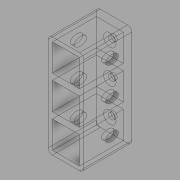
# Autodesk Inventor part: AK-C-C39-Holder
Saved by Autodesk Inventor 2016 (Build 200138000, 138)
## iProperties
Created: 2016-04-02
Part Number: AK-C-C39-Holder
Material: ABS Plastic
Document SubType Name: Modeling
Designer: admin
Density: 1.06 g/cm^3
Appearance: Smooth - White
Author: admin
Autodesk Inventor part; units mm, degrees
ref_plane "YZ Plane" through (0, 0, 0) normal (1, 0, 0) x (0, 1, 0)
ref_plane "XZ Plane" through (0, 0, 0) normal (0, 1, 0) x (-1, 0, 0)
ref_plane "XY Plane" through (0, 0, 0) normal (0, 0, 1) x (1, 0, 0)
derived "AK-C-C39-Main-Board.ipt"
sketch "Sketch2" plane through (0, 0, 0) normal (0, 1, 0) x (-1, 0, 0)
  line L0 (51.25, -29) -> (44, -29)
  line L1 (43.25, -29.75) -> (43.25, -31)
  line L2 (43.25, -31) -> (6.5, -31)
  line L3 (6.5, -31) -> (6.5, -29.75)
  line L4 (5.75, -29) -> (-5.75, -29)
  line L5 (-6.5, -29.75) -> (-6.5, -31)
  line L6 (-6.5, -31) -> (-43.25, -31)
  line L7 (-43.25, -31) -> (-43.25, -29.75)
  line L8 (-44, -29) -> (-51.25, -29)
  line L9 (-51.25, -29) -> (-53.75, -26.5)
  line L10 (-53.75, -26.5) -> (-53.75, -5.5)
  line L11 (-53.75, -5.5) -> (-56.25, -3)
  line L12 (-56.25, -3) -> (-56.25, 18)
  line L13 (-56.25, 18) -> (-54.5, 18)
  line L14 (-53.75, 18.75) -> (-53.75, 26.5)
  line L15 (-53.75, 26.5) -> (-51.25, 29)
  line L16 (-51.25, 29) -> (-44, 29)
  line L17 (-43.25, 29.75) -> (-43.25, 31)
  line L18 (-43.25, 31) -> (-6.5, 31)
  line L19 (-6.5, 31) -> (-6.5, 29.75)
  line L20 (-5.75, 29) -> (5.75, 29)
  line L21 (6.5, 29.75) -> (6.5, 31)
  line L22 (43.25, 31) -> (43.25, 29.75)
  line L23 (43.25, 31) -> (6.5, 31)
  line L24 (44, 29) -> (51.25, 29)
  line L25 (51.25, 29) -> (53.75, 26.5)
  line L26 (53.75, 26.5) -> (53.75, 18.75)
  line L27 (54.5, 18) -> (56.25, 18)
  line L28 (56.25, 18) -> (56.25, -3)
  line L29 (56.25, -3) -> (53.75, -5.5)
  line L30 (53.75, -5.5) -> (53.75, -26.5)
  line L31 (53.75, -26.5) -> (51.25, -29)
  line L32 (44.7, -32.225) -> (5, -32.225)
  line L33 (5, -32.225) -> (5, -29.925)
  line L34 (5, -29.925) -> (3, -29.925)
  line L35 (44.7, -29.925) -> (44.7, -32.225)
  line L36 (46.7, -29.925) -> (44.7, -29.925)
  line L37 (52.7, -29.3928) -> (52.7, -31.925)
  arc A0 (53.5536, -29.0392) -> (52.7, -29.3928) centre (53.2, -29.3928) ccw
  arc A1 (54.9678, -27.125) -> (54.6142, -27.9786) centre (54.9678, -27.625) ccw
  line L38 (55, -17.425) -> (55, -25.125)
  line L39 (0, -20.0068) -> (0, 12.0803) construction
  line L40 (33.1179, 0) -> (-42.957, 0) construction
  line L41 (57.8, 19.125) -> (57.8, -3.3607)
  line L42 (57.8, -3.3607) -> (55, -7.6074)
  line L43 (55.5, 19.125) -> (57.8, 19.125)
  line L44 (55.5, 29.925) -> (49.0175, 23.4425) construction
  line L45 (25.75, -24.5) -> (12.75, -24.5)
  line L46 (12.75, 24.5) -> (25.75, 24.5)
  line L47 (3.3524, -20) -> (-16.6476, -20)
  line L48 (-16.6476, -20) -> (-16.6476, 20)
  line L49 (-16.6476, 20) -> (3.3524, 20)
  line L50 (3.3524, 20) -> (3.3524, -20)
  line L51 (-23.9878, -15) -> (-31.9878, -15) construction
  line L52 (-31.9878, -15) -> (-31.9878, -7) construction
  line L53 (-31.9878, -7) -> (-23.9878, -7) construction
  line L54 (-23.9878, -7) -> (-23.9878, -15) construction
  line L55 (-34.9878, -15) -> (-42.9878, -15) construction
  line L56 (-42.9878, -15) -> (-42.9878, -7) construction
  line L57 (-42.9878, -7) -> (-34.9878, -7) construction
  line L58 (-34.9878, -7) -> (-34.9878, -15) construction
  line L59 (-23.9878, -4) -> (-31.9878, -4) construction
  line L60 (-31.9878, -4) -> (-31.9878, 4) construction
  line L61 (-31.9878, 4) -> (-23.9878, 4) construction
  line L62 (-23.9878, 4) -> (-23.9878, -4) construction
  line L63 (-34.9878, -4) -> (-42.9878, -4) construction
  line L64 (-42.9878, -4) -> (-42.9878, 4) construction
  line L65 (-42.9878, 4) -> (-34.9878, 4) construction
  line L66 (-34.9878, 4) -> (-34.9878, -4) construction
  line L67 (-23.9878, 7) -> (-31.9878, 7) construction
  line L68 (-31.9878, 7) -> (-31.9878, 15) construction
  line L69 (-31.9878, 15) -> (-23.9878, 15) construction
  line L70 (-23.9878, 15) -> (-23.9878, 7) construction
  line L71 (-34.9878, 7) -> (-42.9878, 7) construction
  line L72 (-42.9878, 7) -> (-42.9878, 15) construction
  line L73 (-42.9878, 15) -> (-34.9878, 15) construction
  line L74 (-34.9878, 15) -> (-34.9878, 7) construction
  line L75 (25.75, -22.5) -> (12.75, -22.5) construction
  line L76 (12.75, -22.5) -> (12.75, -9.5) construction
  line L77 (12.75, -9.5) -> (25.75, -9.5) construction
  line L78 (25.75, -9.5) -> (25.75, -22.5) construction
  line L79 (25.75, -6.5) -> (12.75, -6.5) construction
  line L80 (12.75, -6.5) -> (12.75, 6.5) construction
  line L81 (12.75, 6.5) -> (25.75, 6.5) construction
  line L82 (25.75, 6.5) -> (25.75, -6.5) construction
  line L83 (25.75, 9.5) -> (12.75, 9.5) construction
  line L84 (12.75, 9.5) -> (12.75, 22.5) construction
  line L85 (12.75, 22.5) -> (25.75, 22.5) construction
  line L86 (25.75, 22.5) -> (25.75, 9.5) construction
  line L87 (31.9633, -16) -> (17.7262, -16) construction
  line L88 (31.9633, 16) -> (18.8213, 16) construction
  line L89 (19.25, -23.7063) -> (19.25, 24.6931) construction
  arc A2 (10.75, -22.5) -> (12.75, -24.5) centre (12.75, -22.5) ccw
  arc A3 (25.75, -24.5) -> (27.75, -22.5) centre (25.75, -22.5) ccw
  arc A4 (12.75, 24.5) -> (10.75, 22.5) centre (12.75, 22.5) ccw
  arc A5 (27.75, 22.5) -> (25.75, 24.5) centre (25.75, 22.5) ccw
  line L90 (55, -25.125) -> (-54.9956, -25.125) construction
  line L91 (55.5, 25.125) -> (55.5, 23.125)
  line L92 (57.5, 25.125) -> (55.5, 25.125)
  line L93 (-57.5, 25.125) -> (-55.5, 25.125)
  line L94 (-55.5, 25.125) -> (-55.5, 23.125)
  line L95 (-57.5, -25.125) -> (-55, -25.125)
  line L96 (-55, -25.125) -> (-55, -17.425)
  line L97 (55, -25.125) -> (57.5, -25.125)
  line L98 (55.5, 25.125) -> (-55.5, 25.125) construction
  line L99 (48.25, -6.5) -> (48.25, 6.5)
  line L100 (50, -6.5) -> (50, 6.5)
  line L101 (50, -8) -> (48.25, -8)
  line L102 (50, 8) -> (48.25, 8)
  arc A6 (50, -8) -> (50, -6.5) centre (50, -7.25) ccw
  arc A7 (48.25, -6.5) -> (48.25, -8) centre (48.25, -7.25) ccw
  arc A8 (50, 6.5) -> (50, 8) centre (50, 7.25) ccw
  arc A9 (48.25, 8) -> (48.25, 6.5) centre (48.25, 7.25) ccw
  line L103 (-47.75, -6.5) -> (-47.75, 6.5)
  line L104 (-49.5, 8) -> (-47.75, 8)
  line L105 (-49.5, 6.5) -> (-49.5, -6.5)
  line L106 (-49.5, -8) -> (-47.75, -8)
  arc A10 (-47.75, -8) -> (-47.75, -6.5) centre (-47.75, -7.25) ccw
  arc A11 (-49.5, -6.5) -> (-49.5, -8) centre (-49.5, -7.25) ccw
  arc A12 (-47.75, 6.5) -> (-47.75, 8) centre (-47.75, 7.25) ccw
  arc A13 (-49.5, 8) -> (-49.5, 6.5) centre (-49.5, 7.25) ccw
  line L107 (43.75, -27) -> (35.5, -27)
  line L108 (33.75, -27) -> (33.75, -25.25)
  line L109 (35.5, -25.25) -> (43.75, -25.25)
  line L110 (-11, -27) -> (-19.25, -27)
  line L111 (-19.25, -25.25) -> (-11, -25.25)
  line L112 (-9.25, -25.25) -> (-9.25, -27)
  line L113 (-34.25, -27) -> (-44.25, -27)
  line L114 (-44.25, -25.25) -> (-34.25, -25.25)
  line L115 (-44.25, 25.25) -> (-34.25, 25.25)
  line L116 (-34.25, 27) -> (-44.25, 27)
  line L117 (-10.75, 25.25) -> (-19.25, 25.25)
  line L118 (-19.25, 27) -> (-10.75, 27)
  line L119 (-9.25, 27) -> (-9.25, 25.25)
  line L120 (43.75, 25.25) -> (35.25, 25.25)
  line L121 (33.75, 25.25) -> (33.75, 27)
  line L122 (35.25, 27) -> (43.75, 27)
  arc A14 (33.75, -27) -> (35.5, -27) centre (34.625, -27) ccw
  arc A15 (35.5, -25.25) -> (33.75, -25.25) centre (34.625, -25.25) ccw
  arc A16 (-11, -27) -> (-9.25, -27) centre (-10.125, -27) ccw
  arc A17 (-9.25, -25.25) -> (-11, -25.25) centre (-10.125, -25.25) ccw
  arc A18 (33.75, 25.25) -> (35.25, 25.25) centre (34.5, 25.25) ccw
  arc A19 (35.25, 27) -> (33.75, 27) centre (34.5, 27) ccw
  arc A20 (-9.25, 27) -> (-10.75, 27) centre (-10, 27) ccw
  arc A21 (-10.75, 25.25) -> (-9.25, 25.25) centre (-10, 25.25) ccw
  line L123 (27.75, 22.5) -> (27.75, -22.5)
  line L124 (-34.9878, 7) -> (-42.9878, 15) construction
  line L125 (-31.9878, 7) -> (-23.9878, 15) construction
  line L126 (-31.9878, -7) -> (-23.9878, -15) construction
  line L127 (-34.9878, -7) -> (-42.9878, -15) construction
  line L128 (10.75, 7.999) -> (10.75, 8)
  line L129 (10.75, -22.5) -> (10.75, 22.5)
  arc A22 (43.75, 25.25) -> (43.75, 27) centre (43.75, 26.125) ccw
  arc A23 (-19.25, 27) -> (-19.25, 25.25) centre (-19.25, 26.125) ccw
  arc A24 (-34.25, 25.25) -> (-34.25, 27) centre (-34.25, 26.125) ccw
  arc A25 (-44.25, 27) -> (-44.25, 25.25) centre (-44.25, 26.125) ccw
  arc A26 (43.75, -27) -> (43.75, -25.25) centre (43.75, -26.125) ccw
  arc A27 (-19.25, -25.25) -> (-19.25, -27) centre (-19.25, -26.125) ccw
  arc A28 (-34.25, -27) -> (-34.25, -25.25) centre (-34.25, -26.125) ccw
  arc A29 (-44.25, -25.25) -> (-44.25, -27) centre (-44.25, -26.125) ccw
  line L130 (31, 25) -> (29.25, 25)
  line L131 (31, 23.5) -> (31, 20)
  line L132 (29.25, 20) -> (29.25, 23.5)
  arc A30 (31, 23.5) -> (31, 25) centre (31, 24.25) ccw
  arc A31 (29.25, 25) -> (29.25, 23.5) centre (29.25, 24.25) ccw
  arc A32 (29.25, 20) -> (31, 20) centre (30.125, 20) ccw
  line L133 (29.25, -20) -> (29.25, -23.25)
  line L134 (29.25, -25) -> (31, -25)
  line L135 (31, -23.25) -> (31, -20)
  arc A33 (31, -25) -> (31, -23.25) centre (31, -24.125) ccw
  arc A34 (29.25, -23.25) -> (29.25, -25) centre (29.25, -24.125) ccw
  arc A35 (31, -20) -> (29.25, -20) centre (30.125, -20) ccw
  line L136 (9.25, 25) -> (7.5, 25)
  line L137 (7.5, 23.5) -> (7.5, 20)
  line L138 (9.25, 20) -> (9.25, 23.5)
  line L139 (7.5, -20) -> (7.5, -23.25)
  line L140 (7.5, -25) -> (9.25, -25)
  line L141 (9.25, -23.25) -> (9.25, -20)
  arc A36 (9.25, -20) -> (7.5, -20) centre (8.375, -20) ccw
  arc A37 (9.25, -25) -> (9.25, -23.25) centre (9.25, -24.125) ccw
  arc A38 (7.5, -23.25) -> (7.5, -25) centre (7.5, -24.125) ccw
  arc A39 (7.5, 20) -> (9.25, 20) centre (8.375, 20) ccw
  arc A40 (9.25, 23.5) -> (9.25, 25) centre (9.25, 24.25) ccw
  arc A41 (7.5, 25) -> (7.5, 23.5) centre (7.5, 24.25) ccw
  line L142 (29.25, 4) -> (29.25, -4)
  line L143 (31, -4) -> (31, 4)
  line L144 (7.5, 4) -> (7.5, -4)
  line L145 (9.25, -4) -> (9.25, 4)
  arc A42 (31, 4) -> (29.25, 4) centre (30.125, 4) ccw
  arc A43 (29.25, -4) -> (31, -4) centre (30.125, -4) ccw
  arc A44 (9.25, 4) -> (7.5, 4) centre (8.375, 4) ccw
  arc A45 (7.5, -4) -> (9.25, -4) centre (8.375, -4) ccw
  line L146 (-22.75, 30.3253) -> (-30.75, 30.3253) construction
  line L147 (-30.75, 30.3253) -> (-30.75, 22.4164) construction
  line L148 (-30.75, 22.4164) -> (-22.75, 22.4164) construction
  line L149 (-22.75, 22.4164) -> (-22.75, 30.3253) construction
  line L150 (-26.75, 29.9722) -> (-26.75, 20.9797) construction
  arc A46 (6.5, -29.75) -> (5.75, -29) centre (5.75, -29.75) ccw
  arc A47 (-5.75, -29) -> (-6.5, -29.75) centre (-5.75, -29.75) ccw
  arc A48 (-43.25, -29.75) -> (-44, -29) centre (-44, -29.75) ccw
  arc A49 (-54.5, 18) -> (-53.75, 18.75) centre (-54.5, 18.75) ccw
  arc A50 (-44, 29) -> (-43.25, 29.75) centre (-44, 29.75) ccw
  arc A51 (-6.5, 29.75) -> (-5.75, 29) centre (-5.75, 29.75) ccw
  arc A52 (5.75, 29) -> (6.5, 29.75) centre (5.75, 29.75) ccw
  arc A53 (43.25, 29.75) -> (44, 29) centre (44, 29.75) ccw
  arc A54 (53.75, 18.75) -> (54.5, 18) centre (54.5, 18.75) ccw
  arc A55 (44, -29) -> (43.25, -29.75) centre (44, -29.75) ccw
  line L151 (57.5, 27.125) -> (57.5, 25.125)
  line L152 (-57.5, 27.125) -> (-57.5, 25.125)
  point P0 (25.75, -16)
  point P1 (25.75, 16)
  point P2 (19.25, -22.5)
  point P3 (19.25, -24.5)
  point P4 (27.75, 0)
  point P5 (10.75, 0)
  point P6 (-26.75, 30.3253)
  point P7 (-26.75, 18)
  point P8 (-26.75, -18)
  point P9 (-44.75, 0)
sketch "Sketch3" plane through (0, 0, 0) normal (0, 1, 0) x (-1, 0, 0)
  line L0 (55, -25.125) -> (-54.9956, -25.125) construction
  line L1 (55.5, 25.125) -> (-55.5, 25.125) construction
  arc A0 (27.75, 22.5) -> (25.75, 24.5) centre (25.75, 22.5) ccw projected
  line L2 (12.75, 24.5) -> (25.75, 24.5) projected
  arc A1 (12.75, 24.5) -> (10.75, 22.5) centre (12.75, 22.5) ccw projected
  line L3 (10.75, -22.5) -> (10.75, 22.5) projected
  arc A2 (10.75, -22.5) -> (12.75, -24.5) centre (12.75, -22.5) ccw projected
  line L4 (25.75, -24.5) -> (12.75, -24.5) projected
  arc A3 (25.75, -24.5) -> (27.75, -22.5) centre (25.75, -22.5) ccw projected
  line L5 (27.75, 22.5) -> (27.75, -22.5) projected
  point P0 (0, 0)
extrude "Extrusion1" add sketch "Sketch3" along normal blind 4.6
sketch "Sketch4" plane through (0, 4.6, 0) normal (0, 1, 0) x (1, 0, 0)
  line L0 (-55, 25.125) -> (54.9956, 25.125) construction
  line L1 (-55.5, -25.125) -> (55.5, -25.125) construction
  line L2 (-27.75, -22.5) -> (-27.75, 22.5) projected
  arc A0 (-27.75, -22.5) -> (-25.75, -24.5) centre (-25.75, -22.5) ccw projected
  line L3 (-12.75, -24.5) -> (-25.75, -24.5) projected
  arc A1 (-12.75, -24.5) -> (-10.75, -22.5) centre (-12.75, -22.5) ccw projected
  line L4 (-10.75, 22.5) -> (-10.75, -22.5) projected
  arc A2 (-10.75, 22.5) -> (-12.75, 24.5) centre (-12.75, 22.5) ccw projected
  line L5 (-12.75, 24.5) -> (-25.75, 24.5) projected
  arc A3 (-25.75, 24.5) -> (-27.75, 22.5) centre (-25.75, 22.5) ccw projected
  point P0 (0, 0)
extrude "Extrusion2" add sketch "Sketch4" along normal blind 18.4
sketch "Sketch6" plane through (0, 0, 0) normal (0, -1, 0) x (1, 0, 0)
  line L0 (-25.75, 22.5) -> (-25.75, 9.5) projected
  line L1 (-12.75, 22.5) -> (-25.75, 22.5) projected
  line L2 (-12.75, 9.5) -> (-12.75, 22.5) projected
  line L3 (-25.75, 9.5) -> (-12.75, 9.5) projected
  line L4 (-12.75, 6.5) -> (-25.75, 6.5) projected
  line L5 (-25.75, 6.5) -> (-25.75, -6.5) projected
  line L6 (-25.75, -6.5) -> (-12.75, -6.5) projected
  line L7 (-12.75, -6.5) -> (-12.75, 6.5) projected
  line L8 (-12.75, -9.5) -> (-25.75, -9.5) projected
  line L9 (-25.75, -9.5) -> (-25.75, -22.5) projected
  line L10 (-25.75, -22.5) -> (-12.75, -22.5) projected
  line L11 (-12.75, -22.5) -> (-12.75, -9.5) projected
  point P0 (0, 0)
extrude "Extrusion4" cut sketch "Sketch6" against normal blind 21
sketch "Sketch10" plane through (-10.75, 0, 22.5) normal (1, 0, 0) x (0, 0, -1)
  ellipse E0 centre (38.5, 13.5) end of major axis (36.5, 13.5) minor radius 3
  ellipse E1 centre (22.5, 13.5) end of major axis (20.5, 13.5) minor radius 3
  ellipse E2 centre (6.5, 13.5) end of major axis (4.5, 13.5) minor radius 3
  line L0 (45, 23) -> (0, 23)
  line L1 (32, 0) -> (45, 0)
  line L2 (16, 0) -> (29, 0)
  line L3 (0, 0) -> (13, 0)
  point P0 (38.5, 0)
  point P1 (22.5, 0)
  point P2 (6.5, 0)
  dimension "d34" = 3
  dimension "d35" = 2
  dimension "d36" = 3
  dimension "d37" = 2
  dimension "d38" = 3
  dimension "d39" = 2
  dimension "d41" = 9.5
  constraints: 8 end point, 3 midpoint, 3 vertical alignment, 2 horizontal alignment, 6 other
  measures "d41" distance from line of L0 point (6.5, 13.5)
extrude "Extrusion6" cut sketch "Sketch10" against normal through all
sketch "Sketch9" plane through (0, 21, 0) normal (0, -1, 0) x (1, 0, 0)
  line L0 (-31.9633, 16) -> (-18.8213, 16) construction
  line L1 (-19.25, -23.7063) -> (-19.25, 24.6931) construction
  line L2 (-33.1179, 0) -> (42.957, 0) construction
  line L3 (-31.9633, -16) -> (-17.7262, -16) construction
  point P0 (0, 0)
  point P1 (-19.25, 16)
  point P2 (-19.25, 0)
  point P3 (-19.25, -16)
  constraints: 6 point on line
hole "Hole1" at (-19.25, 21, 16) at (-19.25, 21, 0) at (-19.25, 21, -16) direction (0, 1, 0) diameter 3 end through all countersink diameter 6 countersink angle 120
sketch "Sketch5" plane through (0, 23, 0) normal (0, 1, 0) x (1, 0, 0)
  arc A0 (-32.45, -12.75) -> (-32.45, -19.25) centre (-32.45, -16) ccw
  arc A1 (-32.45, 19.25) -> (-32.45, 12.75) centre (-32.45, 16) ccw
  arc A2 (-6.95, -19.25) -> (-6.95, -12.75) centre (-6.95, -16) ccw
  arc A3 (-6.95, 12.75) -> (-6.95, 19.25) centre (-6.95, 16) ccw
  line L0 (-27.2, -24.5) -> (-12.2, -24.5) projected
  arc A4 (-29.2, -22.5) -> (-27.2, -24.5) centre (-27.2, -22.5) ccw projected
  line L1 (-29.2, 22.5) -> (-29.2, -22.5) projected
  arc A5 (-27.2, 24.5) -> (-29.2, 22.5) centre (-27.2, 22.5) ccw projected
  line L2 (-12.2, 24.5) -> (-27.2, 24.5) projected
  arc A6 (-10.2, 22.5) -> (-12.2, 24.5) centre (-12.2, 22.5) ccw projected
  line L3 (-10.2, -22.5) -> (-10.2, 22.5) projected
  arc A7 (-12.2, -24.5) -> (-10.2, -22.5) centre (-12.2, -22.5) ccw projected
  arc A8 (-32.45, 19.25) -> (-29.2, 22.5) centre (-32.45, 22.5) ccw
  arc A9 (-29.2, 9.5) -> (-32.45, 12.75) centre (-32.45, 9.5) ccw
  arc A10 (-6.95, 12.75) -> (-10.2, 9.5) centre (-6.95, 9.5) ccw
  arc A11 (-32.45, -12.75) -> (-29.2, -9.5) centre (-32.45, -9.5) ccw
  arc A12 (-29.2, -22.5) -> (-32.45, -19.25) centre (-32.45, -22.5) ccw
  arc A13 (-10.2, -9.5) -> (-6.95, -12.75) centre (-6.95, -9.5) ccw
  arc A14 (-6.95, -19.25) -> (-10.2, -22.5) centre (-6.95, -22.5) ccw
  arc A15 (-10.2, 22.5) -> (-6.95, 19.25) centre (-6.95, 22.5) ccw
  line L4 (-31.9633, -16) -> (-18.8213, -16) construction
  point P0 (0, 0)
  constraints: 27 point on circle, 20 tangent, 12 centre point, 10 equal radius, 5 point on line, 4 horizontal alignment, 1 end point, 1 vertical alignment
body "Solid1"
